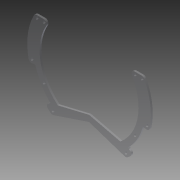
# Autodesk Inventor part: Middle Plate
Saved by Autodesk Inventor 2015 (Build 190159000, 159)
## iProperties
Created: 2016-08-02
Part Number: Middle Plate
Material: Polycarbonate, Clear
Document SubType Name: Modeling
Designer: James Yelland
Density: 1.2 g/cm^3
Appearance: Polycarbonate - Clear
Author: James Yelland
Autodesk Inventor part; units mm, degrees
ref_plane "YZ Plane" through (0, 0, 0) normal (1, 0, 0) x (0, 1, 0)
ref_plane "XZ Plane" through (0, 0, 0) normal (0, 1, 0) x (-1, 0, 0)
ref_plane "XY Plane" through (0, 0, 0) normal (0, 0, 1) x (1, 0, 0)
sketch "Sketch1" plane through (0, 0, 0) normal (0, 1, 0) x (-1, 0, 0)
  circle A0 centre (84.951, 42.5) radius 1.6
  circle A1 centre (93.0625, -19.0886) radius 1.6
  arc A2 (97.9605, -20.0933) -> (89.4144, 44.7534) centre (-0.0036, -0.0174) ccw
  circle A3 centre (73.6122, -42.5) radius 1.6
  circle A4 centre (73.6122, 42.5) radius 1.6
  arc A5 (69.282, -40) -> (69.282, 40) centre (0, 0) ccw
  arc A6 (92.0578, -23.9867) -> (97.9605, -20.0933) centre (93.0625, -19.0886) ccw
  line L0 (93.0625, -19.0886) -> (92.0578, -23.9867) construction
  line L1 (93.0625, -19.0886) -> (97.9605, -20.0933) construction
  arc A7 (77.9423, -45) -> (86.5329, -24.7397) centre (0, 0) ccw
  line L2 (88.8577, -23.3303) -> (92.0578, -23.9867)
  line L3 (84.951, 47.5) -> (73.6122, 47.5)
  arc A8 (73.6122, 47.5) -> (69.282, 40) centre (73.6122, 42.5) ccw
  arc A9 (89.4144, 44.7534) -> (84.951, 47.5) centre (84.951, 42.5) ccw
  arc A10 (88.8577, -23.3303) -> (86.5329, -24.7397) centre (88.4559, -25.2895) ccw
  circle A11 centre (-84.951, 42.5) radius 1.6
  circle A12 centre (-93.0625, -19.0886) radius 1.6
  arc A13 (-89.4144, 44.7534) -> (-97.9605, -20.0933) centre (0.0036, -0.0174) ccw
  circle A14 centre (-73.6122, -42.5) radius 1.6
  circle A15 centre (-73.6122, 42.5) radius 1.6
  arc A16 (-69.282, 40) -> (-69.282, -40) centre (0, 0) ccw
  arc A17 (-97.9605, -20.0933) -> (-92.0578, -23.9867) centre (-93.0625, -19.0886) ccw
  line L4 (-93.0625, -19.0886) -> (-92.0578, -23.9867) construction
  line L5 (-93.0625, -19.0886) -> (-97.9605, -20.0933) construction
  arc A18 (-86.5329, -24.7397) -> (-77.9423, -45) centre (0, 0) ccw
  line L6 (-88.8577, -23.3303) -> (-92.0578, -23.9867)
  line L7 (-84.951, 47.5) -> (-73.6122, 47.5)
  arc A19 (-69.282, 40) -> (-73.6122, 47.5) centre (-73.6122, 42.5) ccw
  arc A20 (-84.951, 47.5) -> (-89.4144, 44.7534) centre (-84.951, 42.5) ccw
  arc A21 (-86.5329, -24.7397) -> (-88.8577, -23.3303) centre (-88.4559, -25.2895) ccw
  arc A22 (66.3816, -74.7896) -> (65.5625, -66.72) centre (63.0625, -71.0502) ccw
  arc A23 (-65.5625, -66.72) -> (-66.3816, -74.7896) centre (-63.0625, -71.0502) ccw
  line L8 (0, -60) -> (-57.4738, -79.1579)
  line L9 (0, -60) -> (57.4738, -79.1579)
  arc A24 (62.1631, -78.3311) -> (66.3816, -74.7896) centre (0, 0) ccw
  arc A25 (-66.3816, -74.7896) -> (-62.1631, -78.3311) centre (0, 0) ccw
  arc A26 (57.4738, -79.1579) -> (62.1631, -78.3311) centre (59.0549, -74.4145) ccw
  arc A27 (-62.1631, -78.3311) -> (-57.4738, -79.1579) centre (-59.0549, -74.4145) ccw
  circle A28 centre (59.0549, -74.4145) radius 1.6
  circle A29 centre (-59.0549, -74.4145) radius 1.6
  arc A30 (64.2173, -63.0566) -> (77.9423, -45) centre (0, 0) ccw
  arc A31 (-77.9423, -45) -> (-64.2173, -63.0566) centre (0, 0) ccw
  line L10 (65.5625, -66.72) -> (64.6443, -66.1899)
  line L11 (-64.6443, -66.1899) -> (-65.5625, -66.72)
  arc A32 (51.2773, -61.4055) -> (69.282, -40) centre (0, 0) ccw
  arc A33 (-69.282, -40) -> (-51.2773, -61.4055) centre (0, 0) ccw
  line L12 (49.5313, -61.8158) -> (0, -50)
  line L13 (-49.5313, -61.8158) -> (0, -50)
  arc A34 (64.2173, -63.0566) -> (64.6443, -66.1899) centre (65.6443, -64.4579) ccw
  arc A35 (-64.6443, -66.1899) -> (-64.2173, -63.0566) centre (-65.6443, -64.4579) ccw
  arc A36 (-51.2773, -61.4055) -> (-49.5313, -61.8158) centre (-49.9954, -59.8704) ccw
  arc A37 (49.5313, -61.8158) -> (51.2773, -61.4055) centre (49.9954, -59.8704) ccw
  point P0 (87.0236, -22.9541)
  point P1 (-87.0236, -22.9541)
  point P2 (71.3525, -70.0629)
  point P3 (86.1122, -20.8494)
  point P4 (-71.3525, -70.0629)
  point P5 (-86.1122, -20.8494)
  point P6 (60, -80)
  point P7 (-60, -80)
  point P8 (62.3749, -64.8797)
  point P9 (-62.3749, -64.8797)
  point P10 (50.4995, -62.0468)
  point P11 (-50.4995, -62.0468)
  dimension "d10" = 3.2
  dimension "d75" = 3.2
  dimension "d77" = 3.2
  dimension "d80" = 90
  dimension "d82" = 2
  dimension "d86" = 5
  dimension "d87" = 3.2
  dimension "d88" = 3.2
  dimension "d89" = 10
  dimension "d90" = 2
  constraints: 64 point on circle, 38 centre point, 28 end point, 14 tangent, 11 coincident, 8 point on line, 4 equal radius
  measures "d10" diameter of A1
  measures "d75" diameter of A3
  measures "d77" diameter of A4
  measures "d80" angle of L0 L1
  measures "d82" radius of A10
  measures "d86" radius of A26
  measures "d87" diameter of A28
  measures "d88" diameter of A29
  measures "d89" distance of L8.start L12.end
  measures "d90" radius of A34
extrude "Extrusion7" add sketch "Sketch1" along normal blind 3
body "Solid3"
